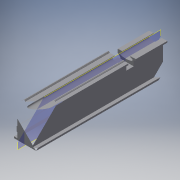
# Autodesk Inventor part: BED
Saved by Autodesk Inventor 2016 (Build 200138000, 138)
## iProperties
Created: 2017-02-14
Part Number: BED
Material: Generic
Document SubType Name: Modeling
Designer: M228540
Density: 1 g/cm^3
Appearance: Default
Author: M228540
Autodesk Inventor part; units mm, degrees
ref_plane "YZ Plane" through (0, 0, 0) normal (1, 0, 0) x (0, 1, 0)
ref_plane "XZ Plane" through (0, 0, 0) normal (0, 1, 0) x (-1, 0, 0)
ref_plane "XY Plane" through (0, 0, 0) normal (0, 0, 1) x (1, 0, 0)
sketch "Sketch1" plane through (0, 0, 0) normal (0, 0, 1) x (1, 0, 0)
  line L0 (11.5951, 4.539) -> (2.0688, 10.039)
  line L1 (11.5951, 4.539) -> (22.5951, 4.539) construction
  line L2 (2.0688, 10.039) -> (-7.9312, 10.039)
  line L3 (-7.9312, 10.039) -> (-7.9312, 21.739)
  line L4 (-7.9312, 21.739) -> (0.168, 31.3911)
  line L5 (0.168, 31.3911) -> (3.968, 31.3911)
  line L6 (3.968, 31.3911) -> (11.7816, 24.8347)
  line L7 (11.7816, 24.8347) -> (11.7816, 21.6347)
  line L8 (11.7816, 21.6347) -> (27.8816, 21.6347)
  line L9 (27.8816, 21.6347) -> (27.8816, 23.6347)
  line L10 (27.8816, 23.6347) -> (53.0816, 23.6347)
  line L11 (53.0816, 23.6347) -> (53.0816, 7.9347)
  line L12 (53.0816, 7.9347) -> (38.3816, 7.9347)
  line L13 (38.3816, 7.9347) -> (38.3816, -0.0653) construction
  line L14 (38.3816, -0.0653) -> (33.7628, -0.0653) construction
  line L15 (38.3816, 7.9347) -> (33.7628, -0.0653)
  line L16 (38.3816, 7.9347) -> (62.019, 7.9347) construction
  line L17 (33.7628, -0.0653) -> (33.7628, -4.0653) construction
  arc A0 (33.7628, -0.0653) -> (29.7628, -4.0653) centre (33.7628, -4.0653) ccw
  line L18 (29.7628, -4.0653) -> (29.7628, -66.0653)
  line L19 (29.7628, -66.0653) -> (29.7628, -270.0653)
  line L20 (-7.9312, 10.039) -> (84.2692, 10.039) construction
  line L21 (-100.1247, 11.1289) -> (-97.9122, 23.6347)
  line L22 (-97.9122, 23.6347) -> (-134.1122, 23.6347)
  line L23 (-97.9122, 23.6347) -> (-61.7122, 23.6347) construction
  line L24 (-134.1122, 23.6347) -> (-134.1122, 21.6347)
  line L25 (-134.1122, 21.6347) -> (-153.1122, 21.6347)
  line L26 (-153.1122, 21.6347) -> (-153.1122, 23.6347)
  line L27 (-153.1122, 23.6347) -> (-161.597, 33.7465)
  line L28 (-161.597, 33.7465) -> (-166.197, 33.7465)
  line L29 (-166.197, 33.7465) -> (-178.4537, 23.4618)
  line L30 (-178.4537, 23.4618) -> (-178.4537, 9.4618)
  line L31 (-178.4537, 9.4618) -> (-164.4537, 9.4618)
  line L32 (-164.4537, 9.4618) -> (-164.4537, 6.4618) construction
  line L33 (-164.4537, 6.4618) -> (-162.7216, 6.4618) construction
  line L34 (-164.4537, 9.4618) -> (-162.7216, 6.4618)
  line L35 (-164.4537, 9.4618) -> (-161.6857, 9.4618) construction
  line L36 (-162.7216, 6.4618) -> (-145.3216, 6.4618)
  line L37 (-145.3216, 6.4618) -> (-145.3216, -16.0382)
  line L38 (-145.3216, -16.0382) -> (-145.3216, -20.5382) construction
  arc A1 (-140.8216, -20.5382) -> (-145.3216, -16.0382) centre (-145.3216, -20.5382) ccw
  line L39 (-140.8216, -20.5382) -> (-140.8216, -156.5382)
  line L40 (-140.8216, -20.5382) -> (-4.8216, -20.5382) construction
  line L41 (-140.8216, -156.5382) -> (-145.3216, -156.5382)
  line L42 (-145.3216, -156.5382) -> (-145.3216, -212.0382)
  line L43 (-145.3216, -212.0382) -> (-140.8216, -211.9963)
  line L44 (-140.8216, -211.9963) -> (-140.2814, -270.0653)
  line L45 (-140.8216, -20.5382) -> (-145.3216, -20.5382) construction
  line L46 (29.7628, -4.0653) -> (33.7628, -4.0653) construction
  line L47 (-140.2814, -270.0653) -> (-175.2814, -270.0653)
  line L48 (-140.2814, -270.0653) -> (-105.2814, -270.0653) construction
  line L49 (-175.2814, -270.0653) -> (-175.2814, -288.0653)
  line L50 (29.7628, -270.0653) -> (64.7628, -270.0653)
  line L51 (29.7628, -270.0653) -> (64.7628, -270.0653) construction
  line L52 (64.7628, -270.0653) -> (64.7628, -288.0653)
  line L53 (64.7628, -288.0653) -> (-175.2814, -288.0653)
  line L54 (-100.1247, 11.1289) -> (-110.7247, 11.1289)
  line L55 (-100.1247, 11.1289) -> (-89.5247, 11.1289) construction
  line L56 (-110.7247, 11.1289) -> (-114.7247, 4.2007)
  line L57 (-114.7247, 4.2007) -> (-119.5652, 1.6273) construction
  line L58 (-119.5652, 1.6273) -> (-124.3686, -3.8711) construction
  line L59 (-124.3686, -3.8711) -> (-125.2529, -14.0346) construction
  line L60 (-125.2529, -14.0346) -> (-112.7247, -24.1844) construction
  line L61 (-112.7247, -24.1844) -> (-52.4666, -30.6089) construction
  line L62 (-52.4666, -30.6089) -> (0.1681, -20.5382) construction
  line L63 (0.1681, -20.5382) -> (13.3927, -13.8206) construction
  line L64 (13.3927, -13.8206) -> (19.8318, -2.7068) construction
  line L65 (19.8318, -2.7068) -> (14.7107, 2.7402) construction
  line L66 (14.7107, 2.7402) -> (11.5951, 4.539) construction
  spline S0 degree 4 poles (-114.7247, 4.2007) (-119.5652, 1.6273) (-124.3686, -3.8711) (-125.2529, -14.0346) (-112.7247, -24.1844) (-52.4666, -30.6089) (0.1681, -20.5382) (13.3927, -13.8206) (19.8318, -2.7068) (14.7107, 2.7402) (11.5951, 4.539) knots 0 0 0 0 0 1 2 3 4 5 6 7 7 7 7 7
  point P0 (0, 0)
  dimension "d0" = 11
  dimension "d1" = 150
  dimension "d2" = 10
  dimension "d3" = 11.7
  dimension "d4" = 12.6
  dimension "d5" = 140
  dimension "d6" = 3.8
  dimension "d7" = 10.2
  dimension "d8" = 140
  dimension "d9" = 3.2
  dimension "d10" = 16.1
  dimension "d11" = 2
  dimension "d12" = 25.2
  dimension "d13" = 15.7
  dimension "d14" = 14.7
  dimension "d15" = 8
  dimension "d16" = 120
  dimension "d17" = 4
  dimension "d18" = 62
  dimension "d19" = 204
  dimension "d22" = 92.2
  dimension "d24" = 12.7
  dimension "d25" = 36.2
  dimension "d26" = 180
  dimension "d27" = 2
  dimension "d28" = 19
  dimension "d29" = 2
  dimension "d30" = 13.2
  dimension "d31" = 140
  dimension "d32" = 4.6
  dimension "d33" = 16
  dimension "d34" = 140
  dimension "d35" = 14
  dimension "d36" = 14
  dimension "d37" = 90
  dimension "d38" = 3
  dimension "d39" = 60
  dimension "d40" = 17.4
  dimension "d41" = 22.5
  dimension "d43" = 136
  dimension "d44" = 90
  dimension "d45" = 4.5
  dimension "d46" = 55.5
  dimension "d47" = 90
  dimension "d50" = 90
  dimension "d51" = 35
  dimension "d52" = 180
  dimension "d53" = 18
  dimension "d54" = 90
  dimension "d55" = 35
  dimension "d57" = 18
  dimension "d58" = 10.6
  dimension "d59" = 180
  dimension "d60" = 8
  dimension "d61" = 120
  dimension "d62" = 62
  dimension "d98" = 4.5
  constraints: 114 end point, 21 perpendicular, 19 horizontal, 6 equal length, 5 vertical, 4 point on circle, 4 point on line, 2 centre point, 2 coincident, 2 parallel, 1 collinear, 3 other
  measures "d0" distance of L0.start L0.end
  measures "d1" angle of L1 L0
  measures "d2" distance of L0.end L2.end
  measures "d3" distance of L2.end L3.end
  measures "d4" distance of L3.end L4.end
  measures "d5" angle of L3 L4
  measures "d6" distance of L4.end L5.end
  measures "d7" distance of L5.end L6.end
  measures "d8" angle of L5 L6
  measures "d9" distance of L6.end L7.end
  measures "d10" distance of L7.end L8.end
  measures "d11" distance of L8.end L9.end
  measures "d12" distance of L9.end L10.end
  measures "d13" distance of L10.end L11.end
  measures "d14" distance of L11.end L12.end
  measures "d15" distance of L12.end L13.end
  measures "d16" angle of L15 L16
  measures "d17" distance of L14.end L17.end
  measures "d18" distance of L18.start L18.end
  measures "d19" distance of L18.end L19.end
  measures "d22" distance of L2.end L21.start
  measures "d24" distance of L21.start L21.end
  measures "d25" distance of L21.end L22.end
  measures "d26" angle of L22 L23
  measures "d27" distance of L22.end L24.end
  measures "d28" distance of L24.end L25.end
  measures "d29" distance of L25.end L26.end
  measures "d30" distance of L26.end L27.end
  measures "d31" angle of L27 L26
  measures "d32" distance of L27.end L28.end
  measures "d33" distance of L28.end L29.end
  measures "d34" angle of L29 L28
  measures "d35" distance of L29.end L30.end
  measures "d36" distance of L30.end L31.end
  measures "d37" angle of L31 L30
  measures "d38" distance of L31.end L32.end
  measures "d39" angle of L34 L35
  measures "d40" distance of L33.end L36.end
  measures "d41" distance of L36.end L37.end
  measures "d43" distance of L39.start L39.end
  measures "d44" angle of L39 L40
  measures "d45" distance of L39.end L41.end
  measures "d46" distance of L41.end L42.end
  measures "d47" angle of L42 L41
  measures "d50" angle of L43 L44
  measures "d51" distance of L44.end L47.end
  measures "d52" angle of L47 L48
  measures "d53" distance of L47.end L49.end
  measures "d54" angle of L49 L47
  measures "d55" distance of L19.end L50.end
  measures "d57" distance of L50.end L52.end
  measures "d58" distance of L21.start L54.end
  measures "d59" angle of L54 L55
  measures "d60" distance of L54.end L56.end
  measures "d61" angle of L56 L54
  measures "d62" distance from line of L5 L61.end
  measures "d98" radius of A1
extrude "Extrusion1" add sketch "Sketch1" against normal blind 1420
chamfer "Chamfer1" distance 4 angle 45 2 edges at (-140.8216, -156.5382, -710) (-140.8216, -211.9963, -710)
ref_plane "Work Plane3" through (-62.686, 23.4618, -1420) normal (-1, 0, 0) x (0, 0, 1)
sketch "Sketch2" plane through (-62.686, 23.4618, -1420) normal (-1, 0, 0) x (0, 0, 1)
  line L0 (1420, 7.9293) -> (0, 7.9293) projected
  line L1 (400, 7.9293) -> (400, -79.7707)
  line L2 (400, -79.7707) -> (318, -79.7707)
  line L3 (318, -79.7707) -> (318, 139.9543)
  line L4 (1420, -27.5272) -> (0, -27.5272) projected
  line L5 (318, 139.9543) -> (400, 139.9543)
  line L6 (400, 139.9543) -> (400, 7.9293)
  line L7 (1420, -27.5272) -> (1420, -293.5272) projected
  point P0 (1420, -23.4618)
  dimension "d68" = 1020
  dimension "d69" = 82
  dimension "d70" = 87.7
  constraints: 10 end point, 4 perpendicular, 2 point on line, 1 vertical
  measures "d68" distance between parallel lines of L7 L1
  measures "d69" distance of L1.end L2.end
  measures "d70" distance between parallel lines of L2 L0
extrude "Extrusion2" cut sketch "Sketch2" along normal through all both and the other way through all
sketch "Sketch3" plane through (0, 0, -1420) normal (0, 0, -1) x (-1, 0, 0)
  line L0 (-11.7816, 21.6347) -> (13.8438, 21.6347)
  line L1 (13.8438, 21.6347) -> (13.8438, 34.9083)
  line L2 (13.8438, 34.9083) -> (-11.7816, 34.9083)
  line L3 (-11.7816, 24.8347) -> (-11.7816, 21.6347) projected
  line L4 (-11.7816, 34.9083) -> (-11.7816, 21.6347)
  point P0 (0, 0)
  constraints: 8 end point, 2 perpendicular, 1 collinear, 1 horizontal
extrude "Extrusion3" cut sketch "Sketch3" against normal up to surface (318 mm away)
sketch "Sketch4" plane through (0, 0, -1420) normal (0, 0, -1) x (-1, 0, 0)
  line L0 (162.7216, 6.4618) -> (145.3216, 6.4618) projected
  line L1 (145.3216, 6.4618) -> (145.3216, 38.0653)
  line L2 (145.3216, 38.0653) -> (188.9756, 38.0653)
  line L3 (188.9756, 38.0653) -> (188.9756, 6.4618)
  line L4 (188.9756, 6.4618) -> (145.3216, 6.4618)
  point P0 (0, 0)
  constraints: 8 end point, 2 perpendicular, 1 collinear, 1 vertical
extrude "Extrusion4" cut sketch "Sketch4" against normal up to surface (318 mm away)
sketch "Sketch5" plane through (0, 0, -1420) normal (0, 0, -1) x (-1, 0, 0)
  arc A0 (145.3216, -16.0382) -> (140.8216, -20.5382) centre (145.3216, -20.5382) ccw projected
  line L0 (143.1229, -16.6119) -> (137.3088, -21.8401) construction
  line L1 (137.3088, -21.8401) -> (131.0577, -25.5382) construction
  line L2 (131.0577, -25.5382) -> (117.2622, -38.2224) construction
  line L3 (117.2622, -38.2224) -> (109.8216, -60.0382) construction
  line L4 (109.8216, -60.0382) -> (113.0606, -81.8001) construction
  line L5 (113.0606, -81.8001) -> (118.0762, -117.7452) construction
  line L6 (118.0762, -117.7452) -> (140.9419, -199.0653) construction
  spline S0 degree 4 poles (143.1229, -16.6119) (137.3088, -21.8401) (131.0577, -25.5382) (117.2622, -38.2224) (109.8216, -60.0382) (113.0606, -81.8001) (118.0762, -117.7452) (140.9419, -199.0653) knots 1 1 1 1 1 2 3 4 5 5 5 5 5
  line L7 (175.2814, -270.0653) -> (140.2814, -270.0653) projected
  line L8 (140.8216, -152.5382) -> (140.8216, -20.5382) projected
  line L9 (140.2814, -270.0653) -> (140.7844, -215.9961) projected
  line L10 (140.9419, -199.0653) -> (140.7844, -215.9961)
  line L11 (140.7844, -215.9961) -> (166.7403, -216.2376)
  line L12 (166.7403, -216.2376) -> (153.1684, -15.9312)
  line L13 (153.1684, -15.9312) -> (143.1229, -16.6119)
  point P0 (0, 0)
  point P1 (141.8818, -156.5627)
  point P2 (141.8818, -211.9923)
  dimension "d77" = 71
  dimension "d78" = 31
  dimension "d79" = 44
  constraints: 8 end point, 2 perpendicular, 1 point on circle, 6 other
  measures "d77" distance from line of L7 L6.end
  measures "d79" vertical distance of A0.start L3.end
extrude "Extrusion5" cut sketch "Sketch5" against normal up to surface (318 mm away) contours L13 L12 L11 L10 S0
sketch "Sketch6" plane through (0, 0, -1420) normal (0, 0, -1) x (-1, 0, 0)
  line L0 (145.3216, 21.6347) -> (134.1122, 21.6347) projected
  line L1 (134.1122, 21.6347) -> (134.1122, 23.6347) projected
  line L2 (134.1122, 23.6347) -> (97.9122, 23.6347) projected
  line L3 (97.9122, 23.6347) -> (100.1247, 11.1289) projected
  line L4 (100.1247, 11.1289) -> (110.7247, 11.1289) projected
  line L5 (110.7247, 11.1289) -> (114.7247, 4.2007) projected
  spline S0 degree 4 poles (114.7247, 4.2007) (119.5652, 1.6273) (124.3686, -3.8711) (125.2529, -14.0346) (112.7247, -24.1844) (52.4666, -30.6089) (-0.1681, -20.5382) (-13.3927, -13.8206) (-19.8318, -2.7068) (-14.7107, 2.7402) (-11.5951, 4.539) knots 0 0 0 0 0 0.142857 0.285714 0.428571 0.571429 0.714286 0.857143 1 1 1 1 1 projected
  line L6 (145.3216, -16.0382) -> (145.3216, 21.6347) projected
  line L7 (-11.5951, 4.539) -> (-2.0688, 10.039) projected
  line L8 (-2.0688, 10.039) -> (7.9312, 10.039) projected
  line L9 (7.9312, 10.039) -> (7.9312, 21.6347) projected
  line L10 (7.9312, 21.6347) -> (-27.8816, 21.6347) projected
  line L11 (-27.8816, 23.6347) -> (-53.0816, 23.6347) projected
  line L12 (-27.8816, 21.6347) -> (-27.8816, 23.6347) projected
  line L13 (-53.0816, 23.6347) -> (-53.0816, 7.9347) projected
  line L14 (-53.0816, 7.9347) -> (-38.3816, 7.9347) projected
  line L15 (-38.3816, 7.9347) -> (-33.7628, -0.0653) projected
  arc A0 (-29.7628, -4.0653) -> (-33.7628, -0.0653) centre (-33.7628, -4.0653) ccw projected
  line L16 (-33.7628, -0.0653) -> (-16.1969, -0.0653)
  line L17 (120.406, -0.0653) -> (145.3216, -0.0653)
  point P0 (0, 0)
  constraints: 4 end point, 2 perpendicular, 2 tangent, 1 point on line, 3 other
extrude "Extrusion6" add sketch "Sketch6" along normal blind 26
sketch "Sketch8" plane through (-145.3216, -16.0382, 0) normal (-1, 0, 0) x (0, 0, 1)
  circle A0 centre (-32.5, 9.5) radius 4
  circle A1 centre (-18.5, 9.5) radius 4
  line L0 (0, 0) -> (0, 22.5) projected
  line L1 (0, 22.5) -> (-1020, 22.5) projected
  point P0 (0, 16.0382)
  dimension "d84" = 8
  dimension "d85" = 8
  dimension "d86" = 18.5
  dimension "d87" = 14
  dimension "d88" = 13
  constraints: 2 centre point, 1 horizontal alignment
  measures "d84" diameter of A1
  measures "d85" diameter of A0
  measures "d86" distance from line of L0 A1.centre
  measures "d87" distance of A1.centre A0.centre
  measures "d88" distance from line of L1 A1.centre
extrude "Extrusion7" cut sketch "Sketch8" against normal blind 10
sketch "Sketch9" plane through (-145.3216, -212.0382, 0) normal (-1, 0, 0) x (0, 0, 1)
  circle A0 centre (-36.5, 33.5) radius 4
  circle A1 centre (-22.5, 33.5) radius 4
  circle A2 centre (-18.5, 205.5) radius 4 projected
  line L0 (0, 0) -> (0, 55.5) projected
  point P0 (0, 212.0382)
  dimension "d91" = 8
  dimension "d92" = 8
  dimension "d93" = 172
  dimension "d94" = 22.5
  dimension "d95" = 14
  constraints: 2 centre point, 1 horizontal alignment
  measures "d91" diameter of A0
  measures "d92" diameter of A1
  measures "d93" vertical distance of A1.centre A2.centre
  measures "d94" distance from line of A1.centre L0
  measures "d95" distance of A1.centre A0.centre
extrude "Extrusion8" cut sketch "Sketch9" against normal blind 20 contours A0 | A1
body "Solid1"
